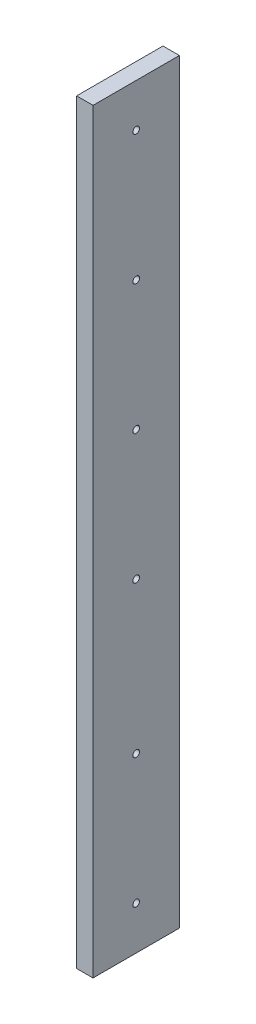
# Autodesk Inventor part: I
Saved by Autodesk Inventor 2024 (Build 280153000, 153)
## iProperties
Created: 2024-03-20
Part Number: I
Material: Generic
Document SubType Name: Modeling
Designer: marco
Density: 1 g/cm^3
Appearance: Wood - Painted White
Author: marco
Autodesk Inventor part; units mm, degrees
ref_plane "YZ Plane" through (0, 0, 0) normal (1, 0, 0) x (0, 1, 0)
ref_plane "XZ Plane" through (0, 0, 0) normal (0, 1, 0) x (-1, 0, 0)
ref_plane "XY Plane" through (0, 0, 0) normal (0, 0, 1) x (1, 0, 0)
sketch "Sketch2" plane through (0, 0, 0) normal (1, 0, 0) x (0, 1, 0)
  line L0 (437.5, -50) -> (-437.5, -50)
  line L1 (-437.5, -50) -> (-437.5, 50)
  line L2 (-437.5, 50) -> (437.5, 50)
  line L3 (437.5, 50) -> (437.5, -50)
  line L4 (437.5, 0) -> (387.5, 0)
  line L5 (87.5, 0) -> (-62.5, 0)
  line L6 (-62.5, 0) -> (-237.5, 0)
  line L7 (-237.5, 0) -> (-387.5, 0)
  line L8 (-387.5, 0) -> (-437.5, 0)
  circle A0 centre (387.5, 0) radius 4
  circle A1 centre (237.5, 0) radius 4
  circle A2 centre (87.5, 0) radius 4
  circle A3 centre (-62.5, 0) radius 4
  circle A4 centre (-237.5, 0) radius 4
  circle A5 centre (-387.5, 0) radius 4
  point P0 (0, 0)
  dimension "d0" = 875
  dimension "d1" = 100
  dimension "d9" = 8
  dimension "d10" = 8
  dimension "d11" = 8
  dimension "d12" = 8
  dimension "d13" = 8
  dimension "d14" = 8
  dimension "d15" = 150
  dimension "d16" = 50
  dimension "d17" = 150
  dimension "d18" = 150
  dimension "d19" = 175
  dimension "d20" = 150
  dimension "d21" = 50
  constraints: 18 end point, 6 centre point, 5 coincident, 2 horizontal, 2 midpoint, 2 parallel, 2 point on line, 1 perpendicular
  measures "d0" distance of L1.end L2.end
  measures "d1" distance of L0.end L1.end
  measures "d9" diameter of A0
  measures "d10" diameter of A1
  measures "d11" diameter of A2
  measures "d12" diameter of A3
  measures "d13" diameter of A4
  measures "d14" diameter of A5
  measures "d15" distance of A1.centre L4.end
  measures "d16" distance of L4.start L4.end
  measures "d17" distance of A2.centre A1.centre
  measures "d18" distance of L5.end L5.start
  measures "d19" distance of L6.end L5.end
  measures "d20" distance of L6.end L7.end
  measures "d21" distance from line of L1 L7.end
extrude "Extrusion1" add sketch "Sketch2" along normal mid plane 19
body "Solid1"
